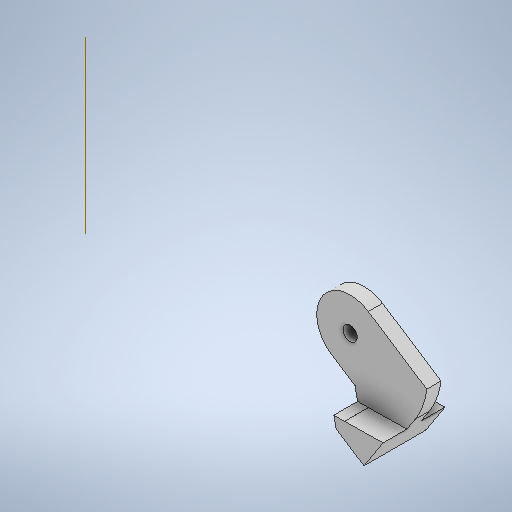
# Autodesk Inventor part: Lock1
Saved by Autodesk Inventor 2025.1 (Build 291241000, 241)
## iProperties
Created: 2026-05-11
Part Number: Lock1
Material: Generic
Document SubType Name: Modeling
Designer: User
Density: 1 g/cm^3
Appearance: Default
Author: User
## iProperties of the stored document Lock1_3DPrint.ipt
Created: 2026-05-12
Part Number: Lock1_3DPrint
Material: Generic
Document SubType Name: Modeling
Designer: User
Density: 1 g/cm^3
Appearance: Default
Author: User
Autodesk Inventor part; units mm, degrees
ref_plane "YZ Plane" through (0, 0, 0) normal (1, 0, 0) x (0, 1, 0)
ref_plane "XZ Plane" through (0, 0, 0) normal (0, 1, 0) x (-1, 0, 0)
ref_plane "Work Plane1" through (0, 0, 0) normal (0, 0, 1) x (1, 0, 0)
sketch "Sketch1" plane through (0, 0, 0) normal (0, 0, 1) x (1, 0, 0)
  circle A0 centre (178.666376, -16.397041) radius 1.5
  line L0 (201.424818, -12.080439) -> (122.055329, -134.544275)
  line L1 (192.303309, -25.235213) -> (190.399763, -28.172305)
  arc A1 (180.569922, -13.459949) -> (176.76283, -19.334134) centre (178.666376, -16.397041) ccw
  line L2 (182.927065, -27.5) -> (174.859284, -22.271227)
  arc A2 (182.473468, -10.522856) -> (174.859284, -22.271227) centre (178.666376, -16.397041) ccw
  line L3 (226.007006, -27.5) -> (182.061376, -27.5)
  line L4 (203.888132, -20.231027) -> (184.377014, -7.585764)
  line L5 (182.473468, -10.522856) -> (194.780372, -18.499029)
  line L6 (180.718486, -30.239399) -> (187.012256, -34.318426)
  arc A3 (192.303309, -25.235213) -> (194.780372, -18.499029) centre (178.666376, -16.397041) ccw
  line L7 (182.622032, -27.302306) -> (180.718486, -30.239399)
  line L8 (192.303309, -25.235213) -> (186.592671, -34.046491)
  point P0 (0, 0)
  point P1 (182.493905, -27.5)
  dimension "d0" = 0.5
  dimension "d1" = 7
  constraints: 14 end point, 6 point on circle, 5 point on line, 3 centre point, 2 coincident, 2 parallel
  measures "d0" distance between parallel lines of L0 L1
  measures "d1" diameter of A1
extrude "Extrusion1" add sketch "Sketch1" along normal blind 3 contours L3 L2 A2 L5 A3 L1 | L1 L8 L6 L7 L3 | L3 L7 L2
sketch "Sketch2" plane through (0, 0, 0) normal (0, 0, -1) x (-1, 0, 0)
  line L0 (-113.222122, -27.5) -> (-151.8, -27.5)
  line L1 (-182.622032, -27.302306) -> (-180.718486, -30.239399)
  line L2 (-180.718486, -30.239399) -> (-186.592671, -34.046491)
  line L3 (-121.635744, -134.27234) -> (-201.005233, -11.808504)
  line L4 (-182.493905, -27.5) -> (-182.493905, -28)
  line L5 (-182.493905, -28) -> (-182.265706, -27.852103)
  line L6 (-182.622032, -27.302306) -> (-180.718486, -30.239399)
  line L7 (-182.493905, -28) -> (-182.169853, -28)
  line L8 (-182.169853, -28) -> (-190.607288, -27.852103)
  point P0 (0, 0)
  point P1 (-182.493905, -27.99432)
  dimension "d10" = 0.5
  constraints: 8 end point, 5 point on line, 2 perpendicular, 1 vertical
  measures "d10" distance of L4.start L4.end
ref_plane "Work Plane2" through (162.2, -27.5, -5) normal (0, 0, -1) x (0, 1, 0)
extrude "Extrusion2" add sketch "Sketch2" along normal up to surface (5 mm away) contours L4 L7 L1 L2 L3 L8
sketch "Sketch3" plane through (0, 0, 3) normal (0, 0, 1) x (1, 0, 0)
  line L0 (190.607288, -27.852103) -> (182.493905, -27.99432)
  line L1 (186.592671, -34.046491) -> (190.607288, -27.852103)
  line L2 (180.718486, -30.239399) -> (186.592671, -34.046491)
  line L3 (182.169853, -28) -> (180.718486, -30.239399)
  line L4 (182.493905, -28) -> (182.169853, -28)
  line L5 (182.493905, -27.99432) -> (182.493905, -28)
  point P0 (0, 0)
extrude "Extrusion3" add sketch "Sketch3" along normal blind 5
chamfer "Chamfer1" distance 3.5 angle 45 1 edges at (182.622, -27.3023, 1.5)
body "Solid1"
